Autodesk Inventor part; units mm, degrees
(part 2 of 2)
  arc A275 (-6.8179, 1.7391) -> (-7.5884, 1.5866) centre (-6.5916, -1.428) ccw
  arc A276 (-6.7356, 2.0348) -> (-6.8179, 1.7391) centre (0, 0) ccw
  arc A277 (-7.3164, 2.5636) -> (-6.7356, 2.0348) centre (-4.905, 4.6292) ccw
  arc A278 (-7.1976, 2.8803) -> (-7.3164, 2.5636) centre (0, 0) ccw
  arc A279 (-6.4123, 2.8966) -> (-7.1976, 2.8803) centre (-6.7395, -0.2617) ccw
  arc A280 (-6.2799, 3.1735) -> (-6.4123, 2.8966) centre (0, 0) ccw
  arc A281 (-6.3164, 3.1678) -> (-6.4308, 2.9286) centre (0, 0) ccw
  arc A282 (-6.4308, 2.9286) -> (-7.219, 2.9074) centre (-6.7395, -0.2617) ccw
  arc A283 (-7.219, 2.9074) -> (-7.3504, 2.5572) centre (0, 0) ccw
  arc A284 (-7.3504, 2.5572) -> (-6.7705, 2.0228) centre (-4.905, 4.6292) ccw
  arc A285 (-6.7705, 2.0228) -> (-6.8416, 1.7674) centre (0, 0) ccw
  arc A286 (-6.8416, 1.7674) -> (-7.6142, 1.6097) centre (-6.5916, -1.428) ccw
  arc A287 (-7.6142, 1.6097) -> (-7.6828, 1.242) centre (0, 0) ccw
  arc A288 (-7.6828, 1.242) -> (-7.0189, 0.8164) centre (-5.6343, 3.7071) ccw
  constraints: 1 coincident, 1 other
extrude "Extrusion5" cut sketch "Sketch12" against normal up to surface (2.5 mm away) contours A1 A2 A3 A4 A5 A6 A7 A8 A28 A29 A30 A31 A33 A56 A58 A46 A47 A54 A51 A50 A49 A63 A65 A93 A91 A89 A88 A85 A84 A103 A98 A99 A101 A120 A121 A122 A123 A124 A125 A126 A127 A128 A156 A157 A158 A159 A160 A161 A162 A163 A225 A226 A227 A228 A229 A230 A231 A232 A273 A274 A275 A276 A277 A278 A279 A280 A257 A258 A259 A260 A261 A262 A263 A264 A241 A242 A243 A244 A245 A246 A247 A248 A207 A208 A209 A210 A211 A212 A213 A214 A215 A190 A191 A192 A193 A194 A195 A196 A197 A172 A173 A174 A175 A176 A177 A178 A179 A180 A138 A139 A140 A141 A142 A143 A144 A145 A146 A104 A105 A106 A107 A108 A109 A110 A111 A66 A67 A68 A69 A70 A71 A72 A73 A74 A43 A45 A41 A39 A18 A20 A22 A25 A27 A0 | A17 A37 A36 A35 A34 A32 A57 A59 A60 A55 A53 A52 A61 A48 A62 A64 A94 A92 A87 A90 A86 A95 A96 A97 A100 A102 A136 A137 A135 A134 A133 A132 A131 A130 A129 A170 A171 A169 A168 A167 A166 A165 A164 A240 A239 A238 A237 A236 A235 A234 A233 A288 A287 A286 A285 A284 A283 A282 A281 A271 A270 A269 A268 A272 A267 A266 A265 A256 A255 A254 A253 A252 A251 A250 A249 A224 A223 A222 A221 A220 A219 A218 A217 A216 A204 A203 A201 A202 A200 A205 A199 A198 A189 A188 A186 A187 A185 A184 A183 A182 A181 A154 A153 A152 A151 A155 A150 A149 A148 A147 A112 A114 A115 A116 A113 A117 A119 A118 A82 A81 A80 A79 A77 A78 A76 A75 A83 A44 A42 A40 A38 A19 A21 A23 A24 A26 A16 A15 A14 A13 A12 A11 A10 A9
body "Solid1"
